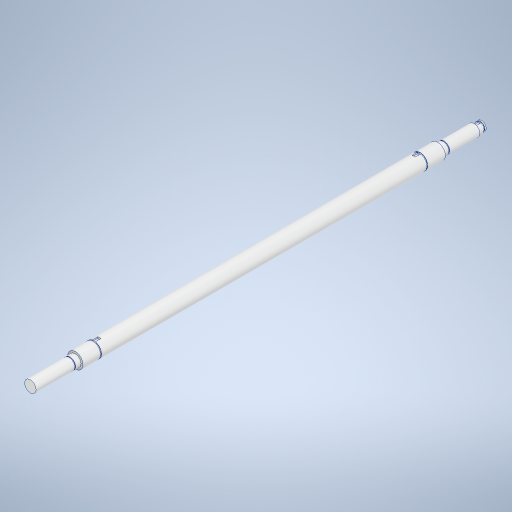
# Autodesk Inventor part: P201
Saved by Autodesk Inventor 2023 (Build 270158000, 158)
## iProperties
Created: 2022-08-29
Part Number: P201
Material: Aluminum 6061
Document SubType Name: Modeling
Designer: D.C. Eksteen
Density: 2.7 g/cm^3
Appearance: Aluminum - Flat
Author: D.C. Eksteen
Title: POWER ROLLER SHAFT
Autodesk Inventor part; units mm, degrees
ref_plane "YZ Plane" through (0, 0, 0) normal (1, 0, 0) x (0, 1, 0)
ref_plane "XZ Plane" through (0, 0, 0) normal (0, 1, 0) x (-1, 0, 0)
ref_plane "XY Plane" through (0, 0, 0) normal (0, 0, 1) x (1, 0, 0)
sketch "Sketch1" plane through (0, 0, 0) normal (1, 0, 0) x (0, 1, 0)
  line L0 (0, 0) -> (7.5, 0)
  line L1 (7.5, 0) -> (7.5, -50)
  line L2 (7.5, -50) -> (7, -50)
  line L3 (7, -50) -> (7, -51.1)
  line L4 (7, -51.1) -> (7.5, -51.1)
  line L5 (7.5, -51.1) -> (7.5, -58.1)
  line L6 (7.5, -58.1) -> (10, -58.1)
  line L7 (10, -58.1) -> (10, -80.8)
  line L8 (10, -80.8) -> (9.5, -80.8)
  line L9 (9.5, -80.8) -> (9.5, -82.1)
  line L10 (9.5, -82.1) -> (10, -82.1)
  line L11 (10, -82.1) -> (10, -502.1)
  line L12 (10, -502.1) -> (9.5, -502.1)
  line L13 (9.5, -502.1) -> (9.5, -503.4)
  line L14 (9.5, -503.4) -> (10, -503.4)
  line L15 (10, -503.4) -> (10, -526.1)
  line L16 (10, -526.1) -> (7.5, -526.1)
  line L17 (7.5, -526.1) -> (7.5, -533.1)
  line L18 (7.5, -533.1) -> (7, -533.1)
  line L19 (7, -533.1) -> (7, -534.2)
  line L20 (7, -534.2) -> (7.5, -534.2)
  line L21 (7.5, -534.2) -> (7.5, -573.1)
  line L22 (7.5, -573.1) -> (0, -573.1)
  line L23 (0, -573.1) -> (0, 0)
  line L24 (6, -573.1) -> (6, -582.9) construction
  line L25 (6, -582.9) -> (0, -582.9)
  line L26 (0, -582.9) -> (0, -573.1)
  line L27 (6, -580.1) -> (5.5, -580.1)
  line L28 (5.5, -580.1) -> (5.5, -581.2)
  line L29 (5.5, -581.2) -> (6, -581.2)
  line L30 (6, -582.9) -> (6, -581.2)
  line L31 (6, -580.1) -> (6, -573.1)
  point P0 (8.75, -526.1)
  point P1 (9.75, -82.1)
  point P2 (9.75, -502.1)
  dimension "d13" = 7.5
  dimension "d14" = 0.5
  dimension "d15" = 50
  dimension "d16" = 1.1
  dimension "d17" = 7
  dimension "d18" = 10
  dimension "d19" = 0.5
  dimension "d20" = 1.3
  dimension "d21" = 1.3
  dimension "d22" = 7.5
  dimension "d23" = 0.5
  dimension "d24" = 1.1
  dimension "d25" = 7
  dimension "d26" = 468
  dimension "d27" = 47
  dimension "d28" = 420
  dimension "d29" = 24
  dimension "d32" = 6
  dimension "d33" = 0.5
  dimension "d34" = 7
  dimension "d35" = 1.1
  dimension "d36" = 1.7
  constraints: 64 end point, 22 perpendicular, 12 point on line, 3 midpoint, 2 collinear, 2 horizontal, 2 vertical
  measures "d13" distance between parallel lines of L23 L1
  measures "d14" distance between parallel lines of L3 L1
  measures "d15" distance between parallel lines of L2 L0
  measures "d16" distance between parallel lines of L4 L2
  measures "d17" distance between parallel lines of L4 L6
  measures "d18" distance between parallel lines of L23 L7
  measures "d19" distance between parallel lines of L9 L7
  measures "d20" distance between parallel lines of L10 L8
  measures "d21" distance between parallel lines of L14 L12
  measures "d22" distance between parallel lines of L23 L17
  measures "d23" distance between parallel lines of L17 L19
  measures "d24" distance between parallel lines of L20 L18
  measures "d25" distance between parallel lines of L16 L18
  measures "d26" distance between parallel lines of L6 L16
  measures "d27" distance from line of point (8.75, -526.1) L22
  measures "d28" distance of point (9.75, -82.1) point (9.75, -502.1)
  measures "d29" distance between parallel lines of L10 L6
  measures "d32" distance between parallel lines of L26 L24
  measures "d33" distance between parallel lines of L28 L24
  measures "d34" distance between parallel lines of L27 L22
  measures "d35" distance between parallel lines of L29 L27
  measures "d36" distance between parallel lines of L25 L29
revolve "Revolution1" add sketch "Sketch1" angle 360 about axis through (0, 0, -573.1) along (0, 0, 1)
sketch "Sketch2" plane through (0, 0, -580.1) normal (0, 0, -1) x (-1, 0, 0)
  circle A0 centre (0, 0) radius 6 projected
  circle A1 centre (0, 0) radius 6 projected
  line L0 (0, 6) -> (2, 6)
  line L1 (2, 6) -> (2, 4)
  line L2 (2, 4) -> (-2, 4)
  line L3 (-2, 4) -> (-2, 6)
  line L4 (-2, 6) -> (0, 6)
  dimension "d37" = 2
  dimension "d38" = 2
  dimension "d39" = 4
  constraints: 10 end point, 4 perpendicular, 2 horizontal, 1 point on line, 1 tangent, 1 vertical alignment, 1 other
  measures "d37" distance of L0.start L0.end
  measures "d38" distance of L0.end L1.end
  measures "d39" distance of L1.end L2.end
extrude "Extrusion1" cut sketch "Sketch2" against normal blind 7 contours L1 L2 L3 A0 | A0 L0 L1 | L3 L4 A0 picked at (0, 4.6667)
sketch "Sketch3" plane through (0, 0, -502.1) normal (0, 0, -1) x (-1, 0, 0)
  circle A0 centre (0, 0) radius 10 projected
  line L0 (0, 10) -> (-2, 10)
  line L1 (-2, 10) -> (-2, 8)
  line L2 (-2, 8) -> (2, 8)
  line L3 (2, 8) -> (2, 10)
  line L4 (2, 10) -> (0, 10)
  point P0 (2, 9.798)
  point P1 (-2, 9.798)
  dimension "d42" = 2
  dimension "d43" = 2
  dimension "d44" = 4
  constraints: 10 end point, 4 perpendicular, 2 horizontal, 1 point on line, 2 other
  measures "d42" distance of L0.start L0.end
  measures "d43" distance of L0.end L1.end
  measures "d44" distance of L1.end L2.end
extrude "Extrusion2" cut sketch "Sketch3" against normal blind 7 contours L3 L2 L1 A0 picked at (0, 8.6667)
sketch "Sketch4" plane through (0, 0, -82.1) normal (0, 0, 1) x (1, 0, 0)
  circle A0 centre (0, 0) radius 10 projected
  line L0 (0, 10) -> (-2, 10)
  line L1 (-2, 8) -> (-2, 9.2871) projected
  line L2 (-2, 10) -> (-2, 8)
  line L3 (2, 8) -> (-2, 8) projected
  line L4 (-2, 8) -> (2, 8)
  line L5 (2, 8) -> (2, 10)
  line L6 (2, 10) -> (0, 10)
  point P0 (0, 0)
  point P1 (-2, 9.2871)
  dimension "d47" = 2
  dimension "d48" = 2
  dimension "d49" = 4
  constraints: 10 end point, 2 collinear, 2 horizontal, 1 perpendicular, 1 point on line, 1 vertical alignment, 1 other
  measures "d47" distance of L0.start L0.end
  measures "d48" distance of L0.end L1.start
  measures "d49" distance of L1.start L3.start
extrude "Extrusion3" cut sketch "Sketch4" against normal blind 7 contours L5 L3 L1 L2 A0 | A0 L6 L5 | L2 L0 A0 picked at (0, 8.6667)
body "Solid1"
